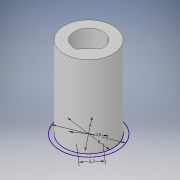
# Autodesk Inventor part: Pieza1
Saved by Autodesk Inventor 2019 (Build 230136000, 136)
## iProperties
Created: 2018-08-28
Part Number: Pieza1
Material: Genérico
Document SubType Name: Modeling
Designer: Cecilia Barrera Vill
Density: 1 g/cm^3
Appearance: Valor por defecto
Author: Cecilia Barrera Vill
Autodesk Inventor part; units mm, degrees
ref_plane "YZ Plane" through (0, 0, 0) normal (1, 0, 0) x (0, 1, 0)
ref_plane "XZ Plane" through (0, 0, 0) normal (0, 1, 0) x (-1, 0, 0)
ref_plane "XY Plane" through (0, 0, 0) normal (0, 0, 1) x (1, 0, 0)
sketch "Boceto1" plane through (0, 0, 0) normal (0, 1, 0) x (-1, 0, 0)
  circle A0 centre (0, 0) radius 1.75
  line L0 (-1.75, 0) -> (-0.2386, 1.7337)
  circle A1 centre (0, 0) radius 3.5
  circle A2 centre (0, 0) radius 3
  circle A3 centre (0, 0) radius 2.5
  dimension "d0" = 3.5
  dimension "d1" = 2.3
  dimension "d2" = 7
  dimension "d5" = 6
  dimension "d8" = 5
  constraints: 4 centre point, 4 coincident, 2 end point, 2 point on circle
  measures "d0" diameter of A0
  measures "d1" distance of L0.start L0.end
  measures "d2" diameter of A1
  measures "d5" diameter of A2
  measures "d8" diameter of A3
extrude "Extrusión1" add sketch "Boceto1" along normal blind 10 contours L0 A0 | A1 | A2 | A3 picked at (-1.2296, 0.716)
extrude "Extrusión2" cut sketch "Boceto1" along normal blind 10 contours A1
